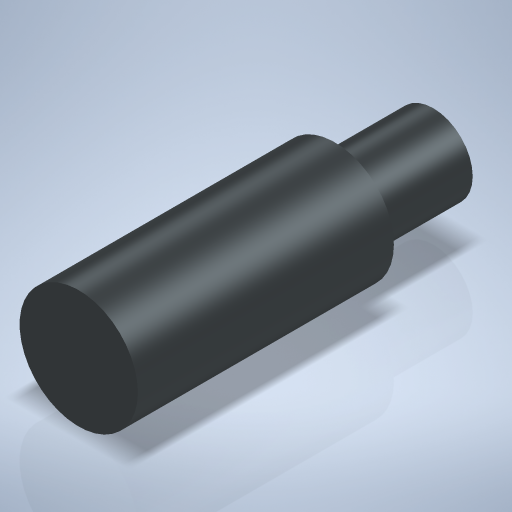
# Autodesk Inventor part: 102 part 3
Saved by Autodesk Inventor 2024 (Build 280153000, 153)
## iProperties
Created: 2024-07-24
Part Number: 102 part 3
Material: Eisen, Guss
Document SubType Name: Modeling
Designer: ffogue
Density: 7.15 g/cm^3
Appearance: Eisen - Grau
Author: ffogue
Autodesk Inventor part; units mm, degrees
ref_plane "YZ Plane" through (0, 0, 0) normal (1, 0, 0) x (0, 1, 0)
ref_plane "XZ Plane" through (0, 0, 0) normal (0, 1, 0) x (-1, 0, 0)
ref_plane "XY Plane" through (0, 0, 0) normal (0, 0, 1) x (1, 0, 0)
sketch "Skizze1" plane through (0, 0, 0) normal (0, 0, 1) x (1, 0, 0)
  line L0 (0, 0) -> (0, 54)
  line L1 (0, 54) -> (6, 54)
  line L2 (6, 54) -> (6, 39)
  line L3 (6, 39) -> (9, 39)
  line L4 (9, 39) -> (9, 0)
  line L5 (9, 0) -> (0, 0)
  point P0 (4.5, 0)
  dimension "d0" = 54
  dimension "d1" = 18
  dimension "d2" = 39
  dimension "d4" = 12
  constraints: 12 end point, 4 perpendicular, 1 horizontal, 1 midpoint, 1 vertical
  measures "d0" distance between parallel lines of L5 L1
  measures "d1" diameter of L4 L0
  measures "d2" distance from line of point (4.5, 0) L3
  measures "d4" diameter of L2 L0
revolve "Umdrehung1" add sketch "Skizze1" angle 360 about axis through (0, 0, 0) along (0, 1, 0)
